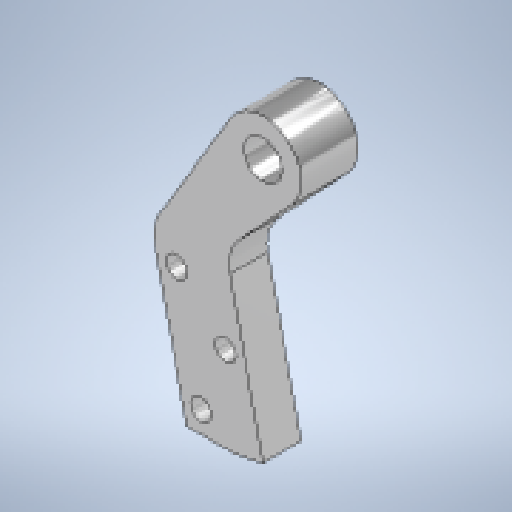
# Autodesk Inventor part: Uprights
Saved by Autodesk Inventor 2023.2 (Build 272271000, 271)
## iProperties
Created: 2024-01-11
Part Number: Uprights
Material: Aluminum 6061
Document SubType Name: Modeling
Designer: Nathan Cai
Mass: 11.7975 g
Surface Area: 25.6985 cm^2
Volume: 4.36943 cm^3
Density: 2.7 g/cm^3
Appearance: Aluminum - Flat
Author: Nathan Cai
Autodesk Inventor part; units mm, degrees
ref_plane "YZ Plane" through (0, 0, 0) normal (1, 0, 0) x (0, 1, 0)
ref_plane "XZ Plane" through (0, 0, 0) normal (0, 1, 0) x (-1, 0, 0)
ref_plane "XY Plane" through (0, 0, 0) normal (0, 0, 1) x (1, 0, 0)
sketch "Sketch3" plane through (0, 0, 0) normal (0, 0, 1) x (1, 0, 0)
  circle A0 centre (0, 0) radius 3.175
  circle A1 centre (0, 0) radius 6.35
  line L0 (-14.4753, -22.7216) -> (-8.2758, -21.3472) construction
  line L1 (-8.2758, -21.3472) -> (-4.1526, -39.9457) construction
  line L2 (-4.1526, -39.9457) -> (-10.3521, -41.3201) construction
  line L3 (-10.3521, -41.3201) -> (-14.4753, -22.7216) construction
  circle A2 centre (-14.4753, -22.7216) radius 1.7526
  circle A3 centre (-6.2142, -30.6464) radius 1.7526
  circle A4 centre (-10.3521, -41.3201) radius 1.7526
  line L4 (-10.3521, -41.3201) -> (-8.2758, -21.3472) construction
  line L5 (-14.4753, -22.7216) -> (-4.1526, -39.9457) construction
  line L6 (0, 0) -> (0, -53.975) construction
  line L7 (-9.3139, -31.3336) -> (-15.4987, -3.436) construction
  line L8 (-15.4987, -3.436) -> (0, 0) construction
  line L9 (-0.0221, -43.9081) -> (-6.2068, -16.0104)
  line L10 (-6.2068, -16.0104) -> (-18.6058, -18.7592)
  line L11 (-18.6058, -18.7592) -> (-12.421, -46.6569)
  line L12 (-12.421, -46.6569) -> (-0.0221, -43.9081)
  line L13 (-0.0221, -43.9081) -> (-18.6058, -18.7592) construction
  line L14 (-6.2068, -16.0104) -> (-12.421, -46.6569) construction
  line L15 (-18.6058, -18.7592) -> (-5.4511, 3.257)
  line L16 (4.6521, -4.322) -> (-6.2068, -16.0104)
  point P0 (-9.3139, -31.3336)
  dimension "d108" = 6.35
  dimension "d109" = 12.7
  dimension "d110" = 19.05
  dimension "d111" = 6.35
  dimension "d112" = 3.5052
  dimension "d113" = 3.5052
  dimension "d114" = 3.5052
  dimension "d115" = 53.975
  dimension "d116" = 12.5
  dimension "d117" = 15.875
  dimension "d118" = 28.575
  dimension "d120" = 12.7
  dimension "d121" = 28.575
  constraints: 34 end point, 5 centre point, 5 midpoint, 5 parallel, 4 coincident, 4 perpendicular, 2 point on circle, 2 tangent, 1 vertical
  measures "d108" diameter of A0
  measures "d109" diameter of A1
  measures "d110" distance between parallel lines of L2 L0
  measures "d111" distance between parallel lines of L3 L1
  measures "d112" diameter of A2
  measures "d113" diameter of A3
  measures "d114" diameter of A4
  measures "d115" distance of L6.start L6.end
  measures "d116" angle of L6 L1
  measures "d117" distance from line of A0.centre L7
  measures "d118" distance from line of point (-9.314, -31.334) L8
  measures "d120" distance of L10.end L9.end
  measures "d121" distance between parallel lines of L12 L10
extrude "Extrusion3" add sketch "Sketch3" along normal blind 6.35
fillet "Fillet5" radius 6.35 2 edges at (-6.2068, -16.0104, 3.175) (-18.6058, -18.7592, 3.175)
chamfer "Chamfer2" distance 7.9375 angle 12.5 1 edges at (-12.421, -46.6569, 3.175) measured on face at (-11.9329, -46.5486, 3.175)
sketch "Sketch4" plane through (0, 0, 0) normal (0, 0, -1) x (-1, 0, 0)
  line L0 (12.8019, -44.9389) -> (4.6717, -44.9389) projected
  line L1 (18.0594, -21.2237) -> (12.8019, -44.9389) projected
  arc A0 (18.0594, -21.2237) -> (17.311, -16.5922) centre (11.86, -19.8493) ccw projected
  line L2 (5.4511, 3.257) -> (17.311, -16.5922) projected
  arc A1 (5.4511, 3.257) -> (-4.6521, -4.322) centre (0, 0) ccw projected
  line L3 (3.938, -13.5683) -> (-4.6521, -4.322) projected
  arc A2 (5.4854, -19.2648) -> (3.938, -13.5683) centre (-0.7141, -17.8904) ccw projected
  line L4 (0.0221, -43.9081) -> (5.4854, -19.2648) projected
  line L5 (4.6717, -44.9389) -> (0.0221, -43.9081) projected
  circle A3 centre (14.4753, -22.7216) radius 1.7526 projected
  circle A4 centre (6.2142, -30.6464) radius 1.7526 projected
  circle A5 centre (10.3521, -41.3201) radius 1.7526 projected
  circle A6 centre (0, 0) radius 3.175 projected
  line L6 (0.0221, -43.9081) -> (5.4854, -19.2648) projected
  line L7 (3.1145, -29.9592) -> (15.5134, -32.708) construction
  line L8 (18.0594, -21.2237) -> (12.8019, -44.9389) projected
  line L9 (18.6058, -18.7592) -> (6.2068, -16.0104)
  line L10 (6.2068, -16.0104) -> (0.0221, -43.9081)
  line L11 (0.0221, -43.9081) -> (12.421, -46.6569)
  line L12 (12.421, -46.6569) -> (18.6058, -18.7592)
  line L13 (18.6058, -18.7592) -> (0.0221, -43.9081) construction
  line L14 (6.2068, -16.0104) -> (12.421, -46.6569) construction
  line L15 (6.2068, -16.0104) -> (5.284, -15.8058)
  arc A7 (5.4854, -19.2648) -> (3.938, -13.5683) centre (-0.7141, -17.8904) ccw projected
  point P0 (9.3139, -31.3336)
  point P1 (18.0949, -18.6459)
  constraints: 16 end point, 5 point on line, 4 perpendicular, 3 midpoint, 2 parallel, 1 point on circle
extrude "Extrusion4" add sketch "Sketch4" along normal blind 3.175 contours L9 L15 A2 L3 A1 L2 A0
chamfer "Chamfer3" distance 7.9375 distance2 3.175 2 edges at (-12.1509, -17.3282, -3.175) (-5.7454, -15.9081, -3.175) measured on face at (-12.2591, -16.84, -3.175) measured on face at (-5.8536, -15.42, -3.175)
body "Solid3"
